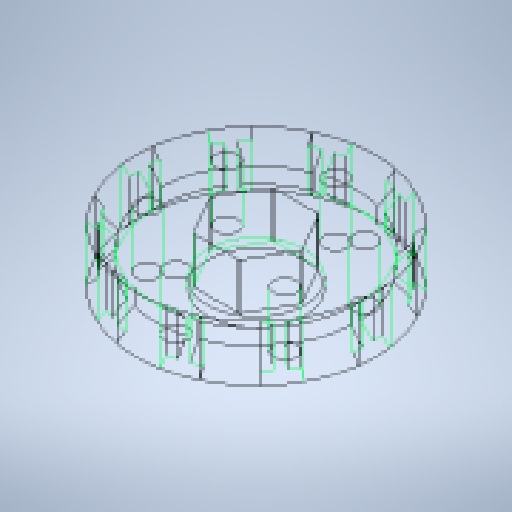
# Autodesk Inventor part: Tire Hub
Saved by Autodesk Inventor 2023.2 (Build 272271000, 271)
## iProperties
Created: 2023-02-06
Part Number: Tire Hub
Material: Nylon 6/6
Document SubType Name: Modeling
Designer: Nathan Cai
Density: 1.13 g/cm^3
Appearance: Smooth - Black
Mass: 9.60807 g
Surface Area: 58.4208 cm^2
Volume: 8.50272 cm^3
Author: Nathan Cai
Autodesk Inventor part; units mm, degrees
ref_plane "YZ Plane" through (0, 0, 0) normal (1, 0, 0) x (0, 1, 0)
ref_plane "XZ Plane" through (0, 0, 0) normal (0, 1, 0) x (-1, 0, 0)
sketch "Sketch1" plane through (0, 0, 0) normal (0, 0, 1) x (1, 0, 0)
  line L0 (0, 12.7) -> (15.875, 12.7)
  line L1 (0, 3.81) -> (15.875, 3.81)
  line L2 (15.875, 12.7) -> (15.875, 3.81)
  line L3 (0, 0) -> (0, 12.7)
  line L4 (0, 12.7) -> (9.525, 12.7)
  line L5 (0, 0) -> (9.525, 0)
  line L6 (9.525, 12.7) -> (0, 12.7)
  line L7 (0, 12.7) -> (0, 0)
  line L8 (9.525, 0) -> (15.875, 0)
  line L9 (15.875, 0) -> (15.875, 3.81)
  line L10 (15.875, 3.81) -> (9.525, 3.81)
  line L11 (15.875, 0) -> (19.05, 3.81)
  line L12 (19.05, 3.81) -> (15.875, 3.81)
  point P0 (0, 3.81)
  dimension "d2" = 15.875
  dimension "d3" = 8.89
  dimension "d5" = 9.525
  dimension "d6" = 12.7
  dimension "d21" = 19.05
  constraints: 26 end point, 6 horizontal, 2 parallel, 2 vertical, 1 perpendicular
  measures "d2" distance of L0.start L0.end
  measures "d3" distance between parallel lines of L1 L0
  measures "d5" distance of L6.end L4.end
  measures "d6" distance between parallel lines of L5 L0
  measures "d21" distance from line of L3 L11.end
revolve "Revolution1" add sketch "Sketch1" angle 360 about axis through (0, 0, 0) along (0, 1, 0) contours L0 L2 L1 L3
sketch "Sketch5" plane through (0, 12.7, 0) normal (0, 1, 0) x (1, 0, 0)
  circle A0 centre (0, 0) radius 19.05
  circle A1 centre (0, 0) radius 15.875
  point P0 (0, 0)
  dimension "d41" = 38.1
  constraints: 2 centre point, 1 coincident, 2 other
  measures "d41" diameter of A0
extrude "Extrusion3" add sketch "Sketch5" against normal blind 3.175
chamfer "Chamfer3" distance 3.175 angle 45 1 edges at (-19.05, 9.525, 0)
ref_plane "Work Plane1" through (0, 8.255, 0) normal (0, -1, 0) x (1, 0, 0)
mirror "Mirror1" about plane through (0, 8.255, 0) normal (0, -1, 0) of "Extrusion3", "Chamfer3"
sketch "Sketch3" plane through (0, 3.81, 0) normal (0, 1, 0) x (1, 0, 0)
  circle A0 centre (0, 0) radius 19.05
  circle A1 centre (0, 0) radius 15.875
  circle A2 centre (0, 0) radius 17.8594
  line L0 (0, 0) -> (-19.0335, 0)
  line L1 (-19.0335, 0) -> (-19.0335, 0.7937) construction
  line L2 (-19.0335, 0.7937) -> (0, 0.7937)
  line L3 (0, 0.7937) -> (0, 0)
  line L4 (-19.0335, -0.7937) -> (0, -0.7937)
  circle A3 centre (0, 0) radius 19.05 projected
  line L5 (-17.7066, 2.3311) -> (-18.887, 2.4865)
  line L6 (-17.7066, -2.3311) -> (-18.887, -2.4865)
  line L7 (-15.8649, -10.5454) -> (-0.4666, 0.6422)
  line L8 (-14.9318, -11.8297) -> (0.4666, -0.6422)
  line L9 (-12.9547, -12.2936) -> (-13.8184, -13.1132)
  line L10 (-15.6951, -8.5218) -> (-16.7415, -9.0899)
  line L11 (-6.6366, -17.8566) -> (-0.7549, 0.2453)
  line L12 (-5.1268, -18.3472) -> (0.7549, -0.2453)
  line L13 (-3.2546, -17.5603) -> (-3.4716, -18.731)
  line L14 (-7.6887, -16.1196) -> (-8.2012, -17.1942)
  line L15 (5.1268, -18.3472) -> (-0.7549, -0.2453)
  line L16 (6.6366, -17.8566) -> (0.7549, 0.2453)
  line L17 (7.6887, -16.1196) -> (8.2012, -17.1942)
  line L18 (3.2546, -17.5603) -> (3.4716, -18.731)
  line L19 (14.9318, -11.8297) -> (-0.4666, -0.6422)
  line L20 (15.8649, -10.5454) -> (0.4666, 0.6422)
  line L21 (15.6951, -8.5218) -> (16.7415, -9.0899)
  line L22 (12.9547, -12.2936) -> (13.8184, -13.1132)
  line L23 (19.0335, -0.7938) -> (0, -0.7937)
  line L24 (19.0335, 0.7937) -> (0, 0.7937)
  line L25 (17.7066, 2.3311) -> (18.887, 2.4865)
  line L26 (17.7066, -2.3311) -> (18.887, -2.4865)
  line L27 (15.8649, 10.5454) -> (0.4666, -0.6422)
  line L28 (14.9318, 11.8297) -> (-0.4666, 0.6422)
  line L29 (12.9547, 12.2936) -> (13.8184, 13.1132)
  line L30 (15.6951, 8.5218) -> (16.7415, 9.0899)
  line L31 (6.6366, 17.8566) -> (0.7549, -0.2453)
  line L32 (5.1268, 18.3472) -> (-0.7549, 0.2453)
  line L33 (3.2546, 17.5603) -> (3.4716, 18.731)
  line L34 (7.6887, 16.1196) -> (8.2012, 17.1942)
  line L35 (-5.1268, 18.3472) -> (0.7549, 0.2453)
  line L36 (-6.6366, 17.8566) -> (-0.7549, -0.2453)
  line L37 (-7.6887, 16.1196) -> (-8.2012, 17.1942)
  line L38 (-3.2546, 17.5603) -> (-3.4716, 18.731)
  line L39 (-14.9318, 11.8297) -> (0.4666, 0.6422)
  line L40 (-15.8649, 10.5454) -> (-0.4666, -0.6422)
  line L41 (-15.6951, 8.5218) -> (-16.7415, 9.0899)
  line L42 (-12.9547, 12.2936) -> (-13.8184, 13.1132)
  point P0 (0, 0)
  point P1 (-13.9677, -11.1293)
  point P2 (-12.3605, -9.9616)
  point P3 (-13.2936, -8.6773)
  point P4 (-14.9008, -9.8449)
  point P5 (-4.7585, -17.2138)
  point P6 (-4.1446, -15.3244)
  point P7 (-5.6544, -14.8339)
  point P8 (-6.2683, -16.7232)
  point P9 (6.2683, -16.7232)
  point P10 (5.6544, -14.8339)
  point P11 (4.1446, -15.3244)
  point P12 (4.7585, -17.2138)
  point P13 (14.9008, -9.8449)
  point P14 (13.2936, -8.6773)
  point P15 (12.3605, -9.9616)
  point P16 (13.9677, -11.1293)
  point P17 (17.8417, 0.7937)
  point P18 (15.8551, 0.7937)
  point P19 (15.8551, -0.7938)
  point P20 (17.8417, -0.7938)
  point P21 (13.9677, 11.1293)
  point P22 (12.3605, 9.9616)
  point P23 (13.2936, 8.6773)
  point P24 (14.9008, 9.8449)
  point P25 (4.7585, 17.2138)
  point P26 (4.1446, 15.3244)
  point P27 (5.6544, 14.8339)
  point P28 (6.2683, 16.7232)
  point P29 (-6.2683, 16.7232)
  point P30 (-5.6544, 14.8339)
  point P31 (-4.1446, 15.3244)
  point P32 (-4.7585, 17.2138)
  point P33 (-14.9008, 9.8449)
  point P34 (-13.2936, 8.6773)
  point P35 (-12.3605, 9.9616)
  point P36 (-13.9677, 11.1293)
  point P37 (-17.8417, -0.7938)
  point P38 (-15.8551, -0.7938)
  point P39 (-15.8551, 0.7937)
  point P40 (-17.8417, 0.7937)
  dimension "d25" = 38.1
  dimension "d27" = 1.1906
  dimension "d26" = 31.75
  dimension "d28" = 0.7937
  dimension "d30" = 7.5
  dimension "d33" = 360
  constraints: 86 end point, 10 point on line, 4 symmetric about line, 3 coincident, 2 parallel, 1 centre point, 1 horizontal, 1 perpendicular, 1 point on circle, 137 other
  measures "d26" diameter of A1
  measures "d28" distance of L0.end L1.end
  measures "d30" angle of L0 L5
extrude "Extrusion2" add sketch "Sketch3" along normal up to surface (8.89 mm away) contours A0 L23 A2 L24 | L24 A2 L25 A0 | A0 L26 A2 L23 | A2 L23 A1 L24 | L30 A2 L27 A0 | A0 L20 A2 L21 | L27 A2 L28 A0 | A1 L28 A2 L27 | A0 L19 A2 L20 | L20 A2 L19 A1 | L28 A2 L29 A0 | A0 L22 A2 L19 | A1 L32 A2 L31 | L16 A2 L15 A1 | L34 A2 L31 A0 | A2 L32 A0 L31 | A0 L16 A2 L17 | L16 A0 L15 A2 | A1 L36 A2 L35 | A2 L33 A0 L32 | L12 A2 L11 A1 | L15 A0 L18 A2 | L35 A0 L38 A2 | A2 L36 A0 L35 | L12 A0 L11 A2 | A2 L13 A0 L12 | A1 L40 A2 L39 | A2 L37 A0 L36 | L8 A2 L7 A1 | L11 A0 L14 A2 | L39 A0 L42 A2 | A2 L40 A0 L39 | L8 A0 L7 A2 | A2 L9 A0 L8 | A1 L0 A2 L2 | A2 L41 A0 L40 | A1 L4 A2 L0 | L7 A0 L10 A2 | L2 A0 L5 A2 | A2 L4 A0 L2 | A2 L6 A0 L4
sketch "Sketch6" plane through (0, 3.81, 0) normal (0, -1, 0) x (1, 0, 0)
  line L0 (0, 0) -> (9.525, 0) construction
  circle A0 centre (0, 0) radius 9.525 projected
  line L1 (7.3323, 0) -> (3.6662, -6.35)
  line L2 (3.6662, -6.35) -> (-3.6662, -6.35)
  line L3 (-3.6662, -6.35) -> (-7.3323, 0)
  line L4 (-7.3323, 0) -> (-3.6662, 6.35)
  line L5 (-3.6662, 6.35) -> (3.6662, 6.35)
  line L6 (3.6662, 6.35) -> (7.3323, 0)
  dimension "d47" = 12.7
  constraints: 14 end point, 1 coincident, 1 horizontal, 1 horizontal alignment, 1 point on line, 14 other
  measures "d47" distance between parallel lines of L5 L2
extrude "Extrusion4" cut sketch "Sketch6" against normal through all contours L1 L2 L3 L4 L5 L6
sketch "Sketch7" plane through (0, 3.81, 0) normal (0, -1, 0) x (1, 0, 0)
  circle A0 centre (0, 0) radius 7.747
  dimension "d50" = 15.494
  constraints: 1 centre point, 1 coincident
  measures "d50" diameter of A0
extrude "Extrusion5" cut sketch "Sketch7" against normal blind 1.524
fillet "Fillet3" radius 0.508 6 edges at (3.6662, 9.017, -6.35) (-3.6662, 9.017, -6.35) (-7.3323, 9.017, 0) (7.3323, 9.017, 0) (3.6662, 9.017, 6.35) (-3.6662, 9.017, 6.35)
sketch "Sketch9" plane through (0, 3.81, 0) normal (0, -1, 0) x (1, 0, 0)
  circle A0 centre (0, 0) radius 12.7 construction
  circle A1 centre (10.9985, 6.35) radius 1.7526
  line L0 (0, 0) -> (12.7, 0) construction
  line L1 (0, 0) -> (10.9985, 6.35) construction
  dimension "d62" = 25.4
  dimension "d63" = 3.5052
  dimension "d76" = 30
  constraints: 4 end point, 2 centre point, 2 point on circle, 1 coincident, 1 horizontal
  measures "d62" diameter of A0
  measures "d63" diameter of A1
  measures "d76" angle of L0 L1
extrude "Extrusion7" cut sketch "Sketch9" against normal blind 25.4
pattern_circular "Circular Pattern1" count 6 over 360 about axis through (0, 3.81, 0) along (0, 1, 0) of "Extrusion7"
body "Solid1"
